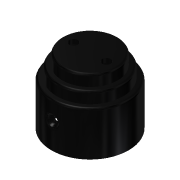
# Autodesk Inventor part: Carcasa
Saved by Autodesk Inventor 2013 SP2 (Build 170200200, 200)
## iProperties
Created: 2014-01-10
Part Number: Carcasa
Material: Generic
Document SubType Name: Modeling
Designer: Koky
Density: 1 g/cm^3
Author: Koky
Autodesk Inventor part; units mm, degrees
sketch "Sketch1" plane through (0, 0, 0) normal (0, 0, 1) x (1, 0, 0)
  point P0 (0, 0)
sketch "Sketch2" plane through (0, 0, 0) normal (0, 0, 1) x (1, 0, 0)
  circle A0 centre (0, 0) radius 35
  dimension "d0" = 70
  constraints: 1 centre point, 1 coincident
  measures "d0" diameter of A0
ref_plane "Work Plane1" through (0, 0, 30) normal (0, 0, 1) x (1, 0, 0)
sketch "Sketch3" plane through (0, 0, 30) normal (0, 0, 1) x (1, 0, 0)
  circle A0 centre (0, 0) radius 30
  dimension "d3" = 60
  constraints: 1 centre point, 1 coincident
  measures "d3" diameter of A0
ref_plane "Work Plane2" through (0, 0, 35) normal (0, 0, 1) x (1, 0, 0)
sketch "Sketch4" plane through (0, 0, 35) normal (0, 0, 1) x (1, 0, 0)
  circle A0 centre (0, 0) radius 25
  dimension "d7" = 50
  constraints: 1 centre point, 1 coincident
  measures "d7" diameter of A0
extrude "Extrusion1" add sketch "Sketch2" along normal blind 40
fillet "Fillet2" radius 2 1 edges at (-35, 0, 40)
ref_plane "Work Plane3" through (0, 0, 40) normal (0, 0, 1) x (1, 0, 0)
sketch "Sketch9" plane through (0, 0, 40) normal (0, 0, 1) x (1, 0, 0)
  circle A0 centre (0, 0) radius 33 projected
  circle A1 centre (0, 0) radius 30
  dimension "d42" = 60
  constraints: 1 centre point, 1 coincident
  measures "d42" diameter of A1
extrude "Extrusion8" add sketch "Sketch9" along normal blind 10 contours A1
sketch "Sketch10" plane through (0, 0, 50) normal (0, 0, 1) x (1, 0, 0)
  circle A0 centre (0, 0) radius 30 projected
  circle A1 centre (0, 0) radius 25
  dimension "d45" = 50
  constraints: 1 centre point, 1 coincident
  measures "d45" diameter of A1
extrude "Extrusion9" add sketch "Sketch10" along normal blind 10 contours A1
sketch "Sketch11" plane through (0, 0, 60) normal (0, 0, 1) x (1, 0, 0)
  circle A0 centre (0, 0) radius 25 projected
  circle A1 centre (0, 0) radius 22.5
  dimension "d48" = 45
  constraints: 1 centre point, 1 coincident
  measures "d48" diameter of A1
extrude "Extrusion10" cut sketch "Sketch11" against normal blind 60 contours A1
sketch "Sketch14" plane through (0, 0, 0) normal (0, 0, -1) x (-1, 0, 0)
  circle A0 centre (0, 0) radius 22.5 projected
  circle A1 centre (0, 0) radius 35 projected
  circle A2 centre (0, 0) radius 30
  dimension "d58" = 60
  constraints: 1 centre point, 1 coincident
  measures "d58" diameter of A2
extrude "Extrusion12" cut sketch "Sketch14" against normal blind 36 contours A2
sketch "Sketch15" plane through (0, 0, 36) normal (0, 0, -1) x (-1, 0, 0)
  circle A0 centre (0, 0) radius 22.5 projected
  circle A1 centre (0, 0) radius 30 projected
ref_plane "Work Plane4" through (0, 0, 60) normal (0, 0, 1) x (1, 0, 0)
sketch "Sketch18" plane through (0, 0, 60) normal (0, 0, 1) x (1, 0, 0)
  circle A0 centre (-14.95, 0) radius 3.75
  line L0 (-49, 0) -> (49, 0) projected
  line L1 (0, -49) -> (0, 49) projected
  circle A1 centre (14.95, 0) radius 3.75
  circle A2 centre (0, 0) radius 22.5
  point P0 (22.5, 0)
  point P1 (-11.2, 0)
  point P2 (10.775, 0)
  dimension "d71" = 7.5
  dimension "d78" = 14.95
  dimension "d81" = 45
  constraints: 3 point on line, 2 centre point, 1 coincident, 1 horizontal alignment, 1 symmetric about line, 3 other
  measures "d78" distance of point (0, 0) point (-14.95, 0)
  measures "d81" diameter of A2
extrude "Extrusion16" add sketch "Sketch18" against normal blind 4 contours L0 L1 A2 A0 | A0 L0 A2 L1 | L1 A2 L0 A1 | L0 A1 A2 L1
fillet "Fillet5" radius 2 2 edges at (-30, 0, 50) (-25, 0, 60)
ref_plane "Work Plane5" through (0, -35, 0) normal (0, 1, 0) x (-1, 0, 0)
sketch "Sketch19" plane through (0, -35, 0) normal (0, 1, 0) x (-1, 0, 0)
  line L0 (49, 0) -> (-49, 0)
  line L1 (0, -12) -> (0, 72)
  arc A0 (0, 27.857143) -> (0, 17.857143) centre (0, 22.857143) ccw
  line L2 (0, 27.857143) -> (0, 17.857143)
  point P0 (0, 0)
  dimension "d86" = 10
  constraints: 3 point on line, 2 end point, 2 point on circle, 1 centre point
  measures "d86" diameter of A0
revolve "Revolution1" cut sketch "Sketch19" angle 360 about axis through (0, -35, -10) along (0, 0, 1)
ref_plane "Work Plane6" through (0, -35, 0) normal (0, 1, 0) x (-1, 0, 0)
sketch "Sketch20" plane through (0, -35, 0) normal (0, 1, 0) x (-1, 0, 0)
  line L0 (0, -12) -> (0, 72)
  line L1 (49, 0) -> (-49, 0)
  line L2 (0, 27.857143) -> (0, 17.857143)
  circle A0 centre (0, 22.857143) radius 2
  point P0 (0, 0)
  dimension "d90" = 4
  constraints: 2 end point, 2 vertical alignment, 1 centre point, 1 collinear, 1 midpoint
  measures "d90" diameter of A0
extrude "Extrusion17" cut sketch "Sketch20" along normal blind 10
ref_plane "Work Plane7" through (0, -29, 0) normal (0, 1, 0) x (-1, 0, 0)
sketch "Sketch21" plane through (0, -29, 0) normal (0, 1, 0) x (-1, 0, 0)
  line L0 (-4.85, 27.7) -> (4.85, 27.7)
  line L1 (4.85, 27.7) -> (4.85, 18)
  line L2 (4.85, 18) -> (-4.85, 18)
  line L3 (-4.85, 18) -> (-4.85, 27.7)
  line L4 (-3.35, 26.2) -> (3.35, 26.2)
  line L5 (3.35, 26.2) -> (3.35, 19.5)
  line L6 (3.35, 19.5) -> (-3.35, 19.5)
  line L7 (-3.35, 19.5) -> (-3.35, 26.2)
  line L8 (-35, 0) -> (35, 0) projected
  line L9 (-49, 0) -> (49, 0) projected
  line L10 (49, 0) -> (-49, 0) projected
  line L11 (0, -12) -> (0, 72) projected
  point P0 (0, 0)
  dimension "d99" = 18
  dimension "d101" = 6.7
  dimension "d102" = 1.5
  dimension "d103" = 1.5
  dimension "d104" = 1.5
  dimension "d105" = 6.7
  constraints: 16 end point, 4 parallel, 2 horizontal, 2 perpendicular
  measures "d99" distance between parallel lines of L8 L2
  measures "d101" distance between parallel lines of L4 L6
  measures "d102" distance between parallel lines of L6 L2
  measures "d103" distance between parallel lines of L4 L0
  measures "d104" distance between parallel lines of L7 L3
  measures "d105" distance between parallel lines of L5 L7
extrude "Extrusion18" add sketch "Sketch21" along normal blind 3 and the other way blind 2 contours L0 L11 L4 L7 L6 L2 L3 | L0 L1 L2 L11 L6 L5 L4
fillet "Fillet6" radius 2 2 edges at (-4.9872, -34.6429, 22.8521) (4.9872, -34.6429, 22.8557)
sketch "Sketch22" plane through (0, 0, 18) normal (0, 0, -1) x (-1, 0, 0)
  arc A0 (-4.85, -29.605363) -> (4.85, -29.605363) centre (0, 0) ccw
  line L0 (-4.85, -26) -> (-4.85, -29.605363)
  line L1 (-4.85, -26) -> (4.85, -26)
  line L2 (4.85, -26) -> (4.85, -29.605363)
  line L3 (-4.85, -29.605363) -> (-4.85, -26)
  arc A1 (-4.85, -29.605363) -> (4.85, -29.605363) centre (0, -1.266986) ccw
  constraints: 6 end point, 2 point on circle, 1 centre point, 1 horizontal, 1 parallel, 1 perpendicular
sketch "Sketch22 outline for Extrusion19" plane through (0, 0, 18) normal (0, 0, -1) x (-1, 0, 0)
  line L0 (-4.85, -26) -> (-4.85, -29.605363)
  line L1 (4.85, -26) -> (-4.85, -26)
  line L2 (4.85, -29.605363) -> (4.85, -26)
  arc A0 (-4.85, -29.605363) -> (4.85, -29.605363) centre (0, 0) ccw
extrude "Extrusion19" cut sketch "Sketch22 outline for Extrusion19" against normal blind 2
sketch "Sketch23" plane through (0, -26, 0) normal (0, 1, 0) x (1, 0, 0)
  line L0 (4.85, -20) -> (3.35, -20)
  line L1 (3.35, -20) -> (3.35, -26.2)
  line L2 (3.35, -26.2) -> (-3.35, -26.2)
  line L3 (-3.35, -26.2) -> (-3.35, -20)
  line L4 (-3.35, -20) -> (-4.85, -20)
  line L5 (-4.85, -20) -> (-4.85, -27.7)
  line L6 (-4.85, -27.7) -> (4.85, -27.7)
  line L7 (4.85, -27.7) -> (4.85, -20)
  line L8 (-3.35, -21.72852) -> (3.35, -21.72852)
  line L9 (3.35, -21.72852) -> (3.35, -26.2)
  line L10 (3.35, -26.2) -> (-3.35, -26.2)
  line L11 (-3.35, -26.2) -> (-3.35, -21.72852)
  point P0 (0, 0)
  constraints: 8 end point, 2 parallel, 1 horizontal, 1 perpendicular, 1 point on line
body "Solid1"
